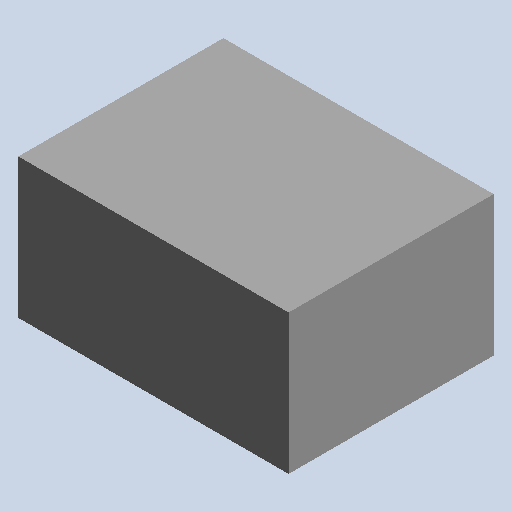
# Autodesk Inventor part: Battery
Saved by Autodesk Inventor 2026 (Build 300175050, 175E)
## iProperties
Part Number: Battery
Material: Generic
Document SubType Name: Modeling
Designer: Kartik
Mass: 1196.25 g
Surface Area: 701.5 cm^2
Volume: 1196.25 cm^3
Density: 1 g/cm^3
Appearance: Default
Author: Kartik
Autodesk Inventor part; units mm, degrees
ref_plane "YZ Plane" through (0, 0, 0) normal (1, 0, 0) x (0, 1, 0)
ref_plane "XZ Plane" through (0, 0, 0) normal (0, 1, 0) x (-1, 0, 0)
ref_plane "XY Plane" through (0, 0, 0) normal (0, 0, 1) x (1, 0, 0)
sketch "Sketch1" plane through (0, 0, 0) normal (0, 0, 1) x (1, 0, 0)
  line L0 (-54.3433, 33.0123) -> (90.6567, 33.0123)
  line L1 (90.6567, 33.0123) -> (90.6567, -41.9877)
  line L2 (90.6567, -41.9877) -> (-54.3433, -41.9877)
  line L3 (-54.3433, -41.9877) -> (-54.3433, 33.0123)
  point P0 (0, 0)
  dimension "d0" = 145
  dimension "d1" = 75
  constraints: 8 end point, 2 parallel, 1 horizontal, 1 perpendicular
  measures "d0" distance of L0.start L0.end
  measures "d1" distance of L2.end L0.start
extrude "Extrusion1" add sketch "Sketch1" along normal blind 110
body "Solid1"
